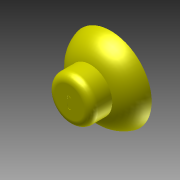
# Autodesk Inventor part: C Stick
Saved by Autodesk Inventor 2012 SP1 (Build 160190100, 190)
## iProperties
Created: 2011-12-19
Part Number: C Stick
Material: Default
Document SubType Name: Modeling
Designer: 133098
Density: 1 g/cm^3
Author: 133098
Autodesk Inventor part; units mm, degrees
ref_plane "YZ Plane" through (0, 0, 0) normal (1, 0, 0) x (0, 1, 0)
ref_plane "XZ Plane" through (0, 0, 0) normal (0, 1, 0) x (-1, 0, 0)
ref_plane "XY Plane" through (0, 0, 0) normal (0, 0, 1) x (1, 0, 0)
sketch "Sketch1" plane through (0, 0, 0) normal (0, 0, 1) x (1, 0, 0)
  circle A0 centre (0, 0) radius 10.795
  dimension "d0" = 21.59
  constraints: 1 centre point, 1 coincident
  measures "d0" diameter of A0
extrude "Extrusion1" add sketch "Sketch1" along normal blind 6.35
fillet "Fillet1" radius 7.62 1 edges at (-10.795, 0, 6.35)
sketch "Sketch2" plane through (0, 0, 0) normal (0, 0, -1) x (-1, 0, 0)
  circle A0 centre (0, 0) radius 10.795 projected
  circle A1 centre (0, 0) radius 5.715
  dimension "d4" = 11.43
  constraints: 1 centre point, 1 coincident
  measures "d4" diameter of A1
extrude "Extrusion2" add sketch "Sketch2" against normal blind 11.43 contours A1
fillet "Fillet2" radius 1.905 1 edges at (5.715, 0, 11.43)
sketch "Sketch3" plane through (0, 0, 11.43) normal (0, 0, 1) x (1, 0, 0)
  line L0 (-0.6917, 1.5054) -> (0.568, 1.5054) construction
  line L1 (0.568, 1.5054) -> (0.568, -1.6512) construction
  line L2 (0.568, -1.6512) -> (-0.6917, -1.6512) construction
  line L3 (-0.6917, -1.6512) -> (-0.6917, 1.5054) construction
  spline S0 degree 2 poles (0.0592, -1.6512) (-0.0915, -1.6512) (-0.3409, -1.4512) (-0.4323, -1.2511) knots 0 0 0 1 2 2 2
  spline S1 degree 2 poles (-0.4323, -1.2511) (-0.5237, -1.0535) (-0.625, -0.4607) (-0.625, -0.0754) knots 0 0 0 1 2 2 2
  spline S2 degree 2 poles (-0.625, -0.0754) (-0.625, 0.3075) (-0.5287, 0.8756) (-0.4348, 1.0855) knots 0 0 0 1 2 2 2
  spline S3 degree 2 poles (-0.4348, 1.0855) (-0.3434, 1.2905) (-0.0939, 1.5054) (0.0617, 1.5054) knots 0 0 0 1 2 2 2
  spline S4 degree 2 poles (0.0617, 1.5054) (0.1382, 1.5054) (0.2741, 1.461) (0.3309, 1.4264) knots 0 0 0 1 2 2 2
  spline S5 degree 2 poles (0.3309, 1.4264) (0.3803, 1.3943) (0.484, 1.3029) (0.5334, 1.2485) knots 0 0 0 1 2 2 2
  line L4 (0.5334, 1.2485) -> (0.5334, 0.7595)
  line L5 (0.5334, 0.7595) -> (0.5162, 0.7595)
  spline S6 degree 2 poles (0.5162, 0.7595) (0.4915, 0.8089) (0.405, 0.9472) (0.3457, 1.0139) knots 0 0 0 1 2 2 2
  spline S7 degree 2 poles (0.3457, 1.0139) (0.2864, 1.0781) (0.1506, 1.1596) (0.0592, 1.1596) knots 0 0 0 1 2 2 2
  spline S8 degree 2 poles (0.0592, 1.1596) (-0.0371, 1.1596) (-0.2125, 0.9991) (-0.2792, 0.8459) knots 0 0 0 1 2 2 2
  spline S9 degree 2 poles (-0.2792, 0.8459) (-0.3434, 0.6903) (-0.415, 0.2186) (-0.415, -0.0754) knots 0 0 0 1 2 2 2
  spline S10 degree 2 poles (-0.415, -0.0754) (-0.415, -0.3891) (-0.3385, -0.8411) (-0.2743, -0.9967) knots 0 0 0 1 2 2 2
  spline S11 degree 2 poles (-0.2743, -0.9967) (-0.21, -1.1474) (-0.0371, -1.3005) (0.0592, -1.3005) knots 0 0 0 1 2 2 2
  spline S12 degree 2 poles (0.0592, -1.3005) (0.1481, -1.3005) (0.2963, -1.2141) (0.3556, -1.1498) knots 0 0 0 1 2 2 2
  spline S13 degree 2 poles (0.3556, -1.1498) (0.4124, -1.0856) (0.4939, -0.9522) (0.5186, -0.9053) knots 0 0 0 1 2 2 2
  line L6 (0.5186, -0.9053) -> (0.5334, -0.9053)
  line L7 (0.5334, -0.9053) -> (0.5334, -1.3894)
  spline S14 degree 2 poles (0.5334, -1.3894) (0.484, -1.4364) (0.3951, -1.5228) (0.3309, -1.5623) knots 0 0 0 1 2 2 2
  spline S15 degree 2 poles (0.3309, -1.5623) (0.2642, -1.6068) (0.1506, -1.6512) (0.0592, -1.6512) knots 0 0 0 1 2 2 2
  constraints: 2 other
extrude "Extrusion3" cut sketch "Sketch3" against normal blind 0.0635
sketch "Sketch4" plane through (0, 0, 0) normal (0, 0, -1) x (-1, 0, 0)
  circle A0 centre (0, 0) radius 10.795 projected
extrude "Extrusion4" cut sketch "Sketch4" against normal blind 0.635
body "Solid1"
